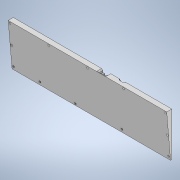
# Autodesk Inventor part: bottom
Saved by Autodesk Inventor 2020 (Build 240168000, 168)
## iProperties
Created: 2019-06-12
Part Number: bottom
Material: Generic
Document SubType Name: Modeling
Designer: Holt
Density: 1 g/cm^3
Appearance: Default
Author: Holt
Autodesk Inventor part; units mm, degrees
ref_plane "YZ Plane" through (0, 0, 0) normal (1, 0, 0) x (0, 1, 0)
ref_plane "XZ Plane" through (0, 0, 0) normal (0, 1, 0) x (-1, 0, 0)
ref_plane "XY Plane" through (0, 0, 0) normal (0, 0, 1) x (1, 0, 0)
sketch "Sketch1" plane through (0, 0, 0) normal (0, 0, 1) x (1, 0, 0)
  line L0 (258.555, 101.5933) -> (258.555, 105.5933)
  line L1 (258.555, 105.5933) -> (0, 105.5933)
  line L2 (0, 105.5933) -> (0, 0)
  line L3 (0, 0) -> (381.837, 0)
  line L4 (381.837, 0) -> (381.837, 105.5933)
  line L5 (381.837, 105.5933) -> (269.555, 105.5933)
  line L6 (269.555, 105.5933) -> (269.555, 101.5933)
  circle A0 centre (190.9185, 101.5933) radius 1.1
  circle A1 centre (67.6763, 7) radius 1.1
  circle A2 centre (152.7499, 4) radius 1.1
  circle A3 centre (378.9641, 53.7131) radius 1.1
  circle A4 centre (3.9928, 7) radius 1.1
  circle A5 centre (377.837, 7) radius 1.1
  circle A6 centre (377.837, 101.5933) radius 1.1
  circle A7 centre (4, 101.5933) radius 1.1
  circle A8 centre (3.9928, 53.7131) radius 1.1
  circle A9 centre (265.3034, 7) radius 1.1
  circle A10 centre (97.459, 101.5933) radius 1.1
  circle A11 centre (277.9185, 101.5933) radius 1.1
  line L7 (258.555, 105.5933) -> (269.555, 105.5933)
  point P0 (0, 0)
  dimension "d53" = 381.837
  dimension "d54" = 105.5933
  dimension "d55" = 105.5933
  dimension "d56" = 2.2
  dimension "d57" = 2.2
  dimension "d58" = 2.2
  dimension "d59" = 2.2
  dimension "d60" = 2.2
  dimension "d61" = 2.2
  dimension "d62" = 2.2
  dimension "d63" = 2.2
  dimension "d64" = 2.2
  dimension "d65" = 2.2
  dimension "d66" = 2.2
  dimension "d67" = 2.2
  constraints: 16 end point, 12 centre point, 1 horizontal
  measures "d53" distance of L2.end L3.end
  measures "d54" distance of L1.end L2.end
  measures "d55" distance of L3.end L4.end
  measures "d56" diameter of A6
  measures "d57" diameter of A11
  measures "d58" diameter of A0
  measures "d59" diameter of A10
  measures "d60" diameter of A7
  measures "d61" diameter of A8
  measures "d62" diameter of A4
  measures "d63" diameter of A1
  measures "d64" diameter of A2
  measures "d65" diameter of A9
  measures "d66" diameter of A5
  measures "d67" diameter of A3
extrude "Extrusion1" add sketch "Sketch1" along normal blind 20
sketch "Sketch5" plane through (0, 0, 0) normal (-1, 0, 0) x (0, 0, 1)
  line L0 (0, 0) -> (20, 0) projected
  line L1 (0, 105.5933) -> (0, 0) projected
  line L2 (3, 0) -> (12.2382, 105.5933)
  line L3 (0, 105.5933) -> (20, 105.5933) projected
  line L4 (20, 105.5933) -> (20, 0) projected
  dimension "d12" = 3
  dimension "d13" = 5
  constraints: 2 end point, 2 point on line
  measures "d12" distance from line of L1 L2.start
  measures "d13" angle of L1 L2
extrude "Extrusion4" cut sketch "Sketch5" against normal through all contours L2 L3 L4 L0
sketch "Sketch6" plane through (0, 0, 0) normal (0, 0, -1) x (-1, 0, 0)
  line L0 (-165.635, 90.4033) -> (-151.635, 90.4033)
  line L1 (-151.635, 90.4033) -> (-151.635, 68.4033)
  line L2 (-151.635, 68.4033) -> (-165.635, 68.4033)
  line L3 (-165.635, 68.4033) -> (-165.635, 90.4033)
  line L4 (-381.837, 0) -> (-381.837, 105.5933) projected
  line L5 (-381.837, 105.5933) -> (0, 105.5933) projected
  line L6 (0, 105.5933) -> (0, 0) projected
  dimension "d16" = 14
  dimension "d17" = 22
  dimension "d19" = 15.19
  dimension "d22" = 151.635
  constraints: 8 end point, 2 parallel, 1 horizontal, 1 perpendicular
  measures "d16" distance of L1.end L2.end
  measures "d17" distance of L0.end L1.end
  measures "d19" distance between parallel lines of L5 L0
  measures "d22" distance between parallel lines of L6 L1
extrude "Extrusion5" cut sketch "Sketch6" against normal blind 2
sketch "Sketch7" plane through (0, 0, 0) normal (0, 0, -1) x (-1, 0, 0)
  line L0 (-193.11, 93.9633) -> (-176.46, 93.9633)
  line L1 (-176.46, 93.9633) -> (-176.46, 84.8633)
  line L2 (-176.46, 84.8633) -> (-193.11, 84.8633)
  line L3 (-193.11, 84.8633) -> (-193.11, 93.9633)
  line L4 (0, 105.5933) -> (0, 0) projected
  line L5 (-381.837, 105.5933) -> (0, 105.5933) projected
  line L6 (-230.725, 96.9723) -> (-216.725, 96.9723)
  line L7 (-216.725, 96.9723) -> (-216.725, 89.9723)
  line L8 (-216.725, 89.9723) -> (-230.725, 89.9723)
  line L9 (-230.725, 89.9723) -> (-230.725, 96.9723)
  line L10 (-297.735, 90.5633) -> (-286.135, 90.5633)
  line L11 (-286.135, 78.6633) -> (-297.735, 78.6633)
  line L12 (-297.735, 78.6633) -> (-297.735, 90.5633)
  line L13 (-286.135, 78.6633) -> (-276.135, 78.6633)
  line L14 (-276.135, 78.6633) -> (-276.135, 90.5633)
  line L15 (-276.135, 90.5633) -> (-286.135, 90.5633)
  dimension "d23" = 16.65
  dimension "d24" = 9.1
  dimension "d25" = 176.46
  dimension "d26" = 11.63
  dimension "d27" = 14
  dimension "d28" = 7
  dimension "d29" = 8.621
  dimension "d30" = 216.725
  dimension "d32" = 11.9
  dimension "d33" = 15.03
  dimension "d51" = 10
  constraints: 28 end point, 5 parallel, 4 horizontal, 4 perpendicular
  measures "d23" distance of L1.end L2.end
  measures "d24" distance of L0.end L1.end
  measures "d25" distance between parallel lines of L4 L1
  measures "d26" distance between parallel lines of L5 L0
  measures "d27" distance of L7.end L8.end
  measures "d28" distance of L6.end L7.end
  measures "d29" distance between parallel lines of L5 L6
  measures "d30" distance between parallel lines of L4 L7
  measures "d32" distance of L10.end L11.start
  measures "d33" distance between parallel lines of L5 L10
  measures "d51" distance of L11.start L13.end
extrude "Extrusion6" cut sketch "Sketch7" against normal blind 4
sketch "Sketch9" plane through (0, 0, 0) normal (0, 0, -1) x (-1, 0, 0)
  line L0 (-370.4105, 63.5933) -> (-370.4105, 103.5933)
  line L1 (-370.4105, 103.5933) -> (-306.4105, 103.5933)
  line L2 (-306.4105, 103.5933) -> (-306.4105, 63.5933)
  line L3 (-306.4105, 63.5933) -> (-370.4105, 63.5933)
  line L4 (-193.11, 84.8633) -> (-193.11, 93.9633) projected
  line L5 (-216.725, 89.9723) -> (-230.725, 89.9723) projected
  line L6 (-381.837, 105.5933) -> (0, 105.5933) projected
  point P0 (0, 0)
  dimension "d44" = 40
  dimension "d45" = 64
  dimension "d52" = 2
  constraints: 8 end point, 2 parallel, 1 perpendicular
  measures "d44" distance of L1.end L2.end
  measures "d45" distance of L0.end L1.end
  measures "d52" distance between parallel lines of L6 L1
extrude "Extrusion8" cut sketch "Sketch9" against normal blind 7
ref_plane "Work Plane1" through (0, 0, 2) normal (0, 0, -1) x (-1, 0, 0)
sketch "Sketch10" plane through (0, 0, 2) normal (0, 0, -1) x (-1, 0, 0)
  circle A0 centre (-3.9928, 7) radius 1.1 projected
  circle A1 centre (-3.9928, 7) radius 2.25
  circle A2 centre (-3.9928, 53.7131) radius 1.1 projected
  circle A3 centre (-3.9928, 53.7131) radius 2.25
  circle A4 centre (-4, 101.5933) radius 1.1 projected
  circle A5 centre (-4, 101.5933) radius 2.25
  circle A6 centre (-97.459, 101.5933) radius 1.1 projected
  circle A7 centre (-97.459, 101.5933) radius 2.25
  circle A8 centre (-190.9185, 101.5933) radius 1.1 projected
  circle A9 centre (-190.9185, 101.5933) radius 2.25
  circle A10 centre (-277.9185, 101.5933) radius 1.1 projected
  circle A11 centre (-277.9185, 101.5933) radius 2.25
  circle A12 centre (-377.837, 101.5933) radius 1.1 projected
  circle A13 centre (-377.837, 101.5933) radius 2.25
  circle A14 centre (-378.9641, 53.7131) radius 1.1 projected
  circle A15 centre (-378.9641, 53.7131) radius 2.25
  circle A16 centre (-377.837, 7) radius 1.1 projected
  circle A17 centre (-377.837, 7) radius 2.25
  circle A18 centre (-265.3034, 7) radius 1.1 projected
  circle A19 centre (-265.3034, 7) radius 2.25
  circle A20 centre (-152.7499, 4) radius 1.1 projected
  circle A21 centre (-152.7499, 4) radius 2.25
  circle A22 centre (-67.6763, 7) radius 1.1 projected
  circle A23 centre (-67.6763, 7) radius 2.25
  point P0 (0, 0)
  dimension "d69" = 4.5
  dimension "d70" = 4.5
  dimension "d71" = 4.5
  dimension "d72" = 4.5
  dimension "d73" = 4.5
  dimension "d74" = 4.5
  dimension "d75" = 4.5
  dimension "d76" = 4.5
  dimension "d77" = 4.5
  dimension "d78" = 4.5
  dimension "d79" = 4.5
  dimension "d80" = 4.5
  constraints: 12 centre point, 12 coincident
  measures "d69" diameter of A1
  measures "d70" diameter of A3
  measures "d71" diameter of A5
  measures "d72" diameter of A7
  measures "d73" diameter of A9
  measures "d74" diameter of A11
  measures "d75" diameter of A13
  measures "d76" diameter of A15
  measures "d77" diameter of A17
  measures "d78" diameter of A19
  measures "d79" diameter of A21
  measures "d80" diameter of A23
extrude "Extrusion9" cut sketch "Sketch10" against normal through all contours A0 | A1 | A2 | A3 | A4 | A5 | A6 | A7 | A8 | A9 | A10 | A11 | A12 | A13 | A14 | A15 | A16 | A17 | A18 | A19 | A20 | A21 | A22 | A23
sketch "Sketch11" plane through (0, 0, 0) normal (0, 0, -1) x (-1, 0, 0)
  line L0 (-269.555, 105.5933) -> (-269.555, 101.5933) projected
  line L1 (-269.555, 105.5933) -> (-269.555, 93.2933)
  line L2 (-258.555, 101.5933) -> (-258.555, 105.5933) projected
  line L3 (-258.555, 105.5933) -> (-258.555, 93.2933)
  line L4 (-269.555, 93.2933) -> (-258.555, 93.2933)
  line L5 (-381.837, 105.5933) -> (0, 105.5933) projected
  point P0 (0, 0)
  dimension "d83" = 12.3
  dimension "d84" = 12.3
  constraints: 6 end point, 1 point on line, 1 vertical
  measures "d83" distance of L0.start L1.end
  measures "d84" distance of L2.end L3.end
extrude "Extrusion10" cut sketch "Sketch11" against normal blind 1.55
fillet "Fillet1" radius 2 3 edges at (269.555, 99.4433, 1.55) (258.555, 97.4433, 1.55) (258.555, 103.5933, 1.55)
sketch "Sketch12" plane through (0, 105.5933, 12.2382) normal (0, 1, 0) x (1, 0, 0)
  line L0 (267.6063, 10.6882) -> (260.5037, 10.6882) projected
  arc A0 (267.6063, 10.6882) -> (269.555, 12.2382) centre (267.6063, 12.6882) ccw projected
  arc A1 (258.555, 12.2382) -> (260.5037, 10.6882) centre (260.5037, 12.6882) ccw projected
  arc A2 (256.6063, 11.7882) -> (260.5037, 8.6882) centre (260.5037, 12.6882) ccw
  line L1 (260.5037, 8.6882) -> (267.6063, 8.6882)
  arc A3 (267.6063, 8.6882) -> (271.5037, 11.7882) centre (267.6063, 12.6882) ccw
  line L2 (271.5037, 11.7882) -> (271.5037, 12.2382)
  line L3 (381.837, 12.2382) -> (269.555, 12.2382) projected
  line L4 (256.6063, 11.7882) -> (256.6063, 12.2382)
  line L5 (258.555, 12.2382) -> (0, 12.2382) projected
  dimension "d88" = 2
  constraints: 6 end point, 4 point on circle, 2 centre point, 2 point on line, 1 parallel, 1 vertical, 2 other
  measures "d88" distance between parallel lines of L0 L1
extrude "Extrusion11" cut sketch "Sketch12" against normal blind 2
sketch "Sketch13" plane through (0, 0, 0) normal (0, 0, -1) x (-1, 0, 0)
  line L0 (0, 105.5933) -> (-381.837, 105.5933) projected
  line L1 (-228.725, 105.5933) -> (-218.725, 105.5933)
  line L2 (-218.725, 105.5933) -> (-218.725, 93.5933)
  line L3 (-218.725, 93.5933) -> (-228.725, 93.5933)
  line L4 (-228.725, 93.5933) -> (-228.725, 105.5933)
  line L5 (0, 105.5933) -> (0, 0) projected
  dimension "d91" = 10
  dimension "d92" = 12
  dimension "d93" = 218.725
  constraints: 8 end point, 2 parallel, 1 horizontal, 1 perpendicular, 1 point on line
  measures "d91" distance of L2.end L3.end
  measures "d92" distance of L1.end L2.end
  measures "d93" distance between parallel lines of L5 L2
extrude "Extrusion12" cut sketch "Sketch13" against normal blind 5.2
move faces "Move1" translate (-2, 0, 0) faces at (228.725, 102.7196, 3.0667)
move faces "Move2" translate (2, 0, 0) faces at (218.725, 102.7196, 3.0667)
move faces "Move3" translate (0, 0, -1.2) faces at (224.725, 101.5933, 5.2)
move faces "Move4" translate (0, 0, -0.805) faces at (222.725, 92.3056, 4)
sketch "Sketch14" plane through (230.725, 89.9723, 3.195) normal (0, 0, -1) x (-1, 0, 0)
  line L0 (0, 7) -> (4, 7) projected
  line L1 (0, 0) -> (0, 7) projected
  line L2 (14, 0) -> (0, 0) projected
  line L3 (14, 7) -> (14, 0) projected
  line L4 (10, 7) -> (14, 7) projected
  line L5 (10, 15.621) -> (10, 7) projected
  line L6 (4, 15.621) -> (10, 15.621) projected
  line L7 (4, 7) -> (4, 15.621) projected
  line L8 (4, 7) -> (10, 7)
  point P0 (230.725, -89.9723)
  constraints: 2 end point, 1 horizontal
extrude "Extrusion13" cut sketch "Sketch14" against normal blind 1 contours L0 L8 L4 L3 L2 L1
sketch "Sketch15" plane through (0, 105.5933, 12.2382) normal (0, 1, 0) x (1, 0, 0)
  line L0 (226.725, 12.2382) -> (226.725, 9.0432) projected
  line L1 (226.725, 9.0432) -> (220.725, 9.0432) projected
  line L2 (220.725, 9.0432) -> (220.725, 12.2382) projected
  line L3 (231.725, 12.2382) -> (231.725, 4.0432)
  line L4 (215.725, 4.0432) -> (215.725, 12.2382)
  line L5 (231.725, 4.0432) -> (215.725, 4.0432)
  line L6 (256.6063, 12.2382) -> (226.725, 12.2382) projected
  line L7 (220.725, 12.2382) -> (0, 12.2382) projected
  dimension "d110" = 5
  dimension "d111" = 5
  dimension "d112" = 5
  constraints: 6 end point, 2 parallel, 1 horizontal
  measures "d110" distance between parallel lines of L0 L3
  measures "d111" distance between parallel lines of L2 L4
  measures "d112" distance between parallel lines of L1 L5
extrude "Extrusion14" cut sketch "Sketch15" against normal blind 7
chamfer "Chamfer2" distance 3 angle 45 3 edges at (231.725, 105.5933, 4.0975) (223.725, 105.5933, 8.195) (215.725, 105.5933, 4.0975)
body "Solid1"
